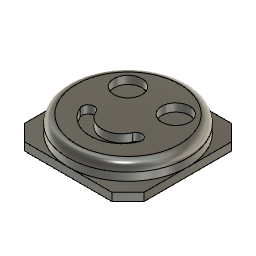
Emoji (Autodesk Fusion 360 design; units mm, degrees)
Autodesk Fusion 360 part; units mm, degrees
sketch "Sketch1" plane through (0, 0, 0) normal (0, 0, 1) x (1, 0, 0)
  line L0 (-75, 75) -> (75, 75)
  line L1 (75, 75) -> (75, -75)
  line L2 (75, -75) -> (-75, -75)
  line L3 (-75, -75) -> (-75, 75)
  line L4 (-75, 75) -> (75, -75) construction
  line L5 (75, 75) -> (-75, -75) construction
  dimension "d1" = 150
  dimension "d2" = 150
  constraint horizontal L0
  constraint perpendicular L0 L1
  constraint parallel L0 L2
  constraint parallel L1 L3
  constraint coincident L4 origin
  constraint coincident L5 origin
  measures "d1" distance of L1.end L2.end
  measures "d2" distance of L0.end L1.end
extrude "Extrude1" add sketch "Sketch1" along normal blind 10
sketch "Sketch2" plane through (0, 0, 10) normal (0, 0, 1) x (-1, 0, 0)
  line L0 (75, 75) -> (-75, 75)
  line L1 (-75, 75) -> (-75, -75)
  line L2 (-75, -75) -> (75, -75)
  line L3 (75, -75) -> (75, 75)
  circle A0 centre (0, 0) radius 75
  constraint coincident A0.centre origin
  constraint tangent L3 A0
extrude "Extrude2" add sketch "Sketch2" along normal blind 20 contours A0
sketch "Sketch3" plane through (0, 0, 30) normal (0, 0, 1) x (-1, 0, 0)
  circle A0 centre (0, 0) radius 75
  circle A1 centre (-30, -30) radius 17.5
  line L0 (0, -2.5) -> (0, -20)
  circle A2 centre (30, -30) radius 17.5
  arc A3 (36.9231, 22.8846) -> (-36.9231, 22.8846) centre (0, 7.5) ccw
  arc A4 (23.0769, 17.1154) -> (36.9231, 22.8846) centre (30, 20) ccw
  arc A5 (23.0769, 17.1154) -> (-23.0769, 17.1154) centre (0, 7.5) ccw
  arc A6 (-36.9231, 22.8846) -> (-23.0769, 17.1154) centre (-30, 20) ccw
  arc A7 (30, 20) -> (-30, 20) centre (0, 7.5) ccw construction
  dimension "d7" = 35
  dimension "d8" = 15
  constraint symmetric A1 L0 A2
  constraint tangent A3 A4
  constraint tangent A4 A5
  constraint tangent A5 A6
  constraint tangent A3 A6
  measures "d7" diameter of A1
  measures "d8" diameter of A6
extrude "Extrude3" cut sketch "Sketch3" against normal blind 10 contours A1 | A2 | A3 A4 A5 A6
chamfer "Chamfer1" distance 20 angle 45 4 edges at (75, 75, 5) (75, -75, 5) (-75, -75, 5) (-75, 75, 5)
fillet "Fillet1" radius 10 1 edges at (69.9246, 27.1212, 30)
